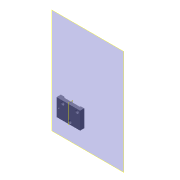
# Autodesk Inventor part: cellSTORM_v5_chiptray_old_0
Saved by Autodesk Inventor 2022 (Build 260153000, 153)
## iProperties
Created: 2020-05-10
Part Number: cellSTORM_v5_chiptray_old_0
Material: Generic
Document SubType Name: Modeling
Designer: diederichbenedict
Density: 1 g/cm^3
Appearance: Default
Author: diederichbenedict
Autodesk Inventor part; units mm, degrees
ref_plane "YZ Plane" through (0, 0, 0) normal (1, 0, 0) x (0, 1, 0)
ref_plane "XZ Plane" through (0, 0, 0) normal (0, 1, 0) x (-1, 0, 0)
ref_plane "XY Plane" through (0, 0, 0) normal (0, 0, 1) x (1, 0, 0)
ref_plane "Work Plane1" through (52.5141, 202.7033, 6.4479) normal (0, 0, -1) x (0, 1, 0)
sketch "Sketch1" plane through (52.5141, 202.7033, 6.4479) normal (0, 0, -1) x (0, 1, 0)
  line L0 (-34.8114, -13.0433) -> (-63.8114, -13.0433)
  line L1 (-63.8114, -13.0433) -> (-63.8114, -52.6244)
  line L2 (-63.8114, -52.6244) -> (-34.8114, -52.6244)
  line L3 (-34.8114, -52.6244) -> (-34.8114, -13.0433)
  circle A0 centre (-59.5444, -32.8338) radius 2.95
  circle A1 centre (-38.8114, -20.7095) radius 2.95
  circle A2 centre (-38.8114, -44.9582) radius 2.95 construction
  line L4 (-60.26, -25.0657) -> (-36.5, -25.0657) construction
  line L5 (-36.5, -25.0657) -> (-36.5, -52.0657) construction
  line L6 (-60.26, -52.0657) -> (-60.26, -25.0657) construction
  line L7 (-57.1632, -22.5233) -> (-33.4032, -22.5233) construction
  line L8 (-33.4032, -22.5233) -> (-33.4032, -49.5233) construction
  line L9 (-33.4032, -49.5233) -> (-57.1632, -49.5233) construction
  line L10 (-57.1632, -49.5233) -> (-57.1632, -22.5233) construction
  circle A3 centre (-38.8114, -44.9582) radius 2.95
  point P0 (-202.7033, -52.5141)
  point P1 (-56.7146, -27.9576)
  point P2 (-25.3114, -32.8338)
  dimension "d4" = 5.9
  dimension "d5" = 5.9
  dimension "d6" = 5.9
  dimension "d37" = 12.1244
  dimension "d38" = 12.1244
  constraints: 22 end point, 5 parallel, 4 centre point, 3 horizontal, 3 perpendicular, 1 coincident, 1 concentric, 1 other
  measures "d4" diameter of A0
  measures "d5" diameter of A1
  measures "d6" diameter of A2
  measures "d37" vertical distance of A1.centre A0.centre
  measures "d38" vertical distance of A2.centre A0.centre
extrude "Extrusion1" add sketch "Sketch1" along normal blind 4
sketch "Sketch2" plane through (52.5141, 202.7033, 2.4479) normal (0, 0, -1) x (-1, 0, 0)
  circle A0 centre (44.9582, -38.8114) radius 2.95 projected
  circle A1 centre (20.7095, -38.8114) radius 2.95 projected
  circle A2 centre (32.8338, -59.5444) radius 2.95 projected
  line L0 (13.0433, -34.8114) -> (13.0433, -63.8114) projected
  line L1 (13.0433, -63.8114) -> (52.6244, -63.8114) projected
  line L2 (52.6244, -63.8114) -> (52.6244, -34.8114) projected
  line L3 (52.6244, -34.8114) -> (13.0433, -34.8114) projected
  point P0 (52.5141, -202.7033)
extrude "Extrusion2" add sketch "Sketch2" along normal blind 1.5 contours A0 | A1 | A2 | L3 L2 L1 L0
sketch "Sketch5" plane through (52.5141, 202.7033, 0.9479) normal (0, 0, -1) x (-1, 0, 0)
  arc A0 (46.5221, -54.1283) -> (46.5221, -43.4579) centre (46.5221, -48.7931) ccw projected
  circle A1 centre (49.353, -48.7931) radius 1.4
  point P0 (52.5141, -202.7033)
  dimension "d30" = 2.8
  constraints: 1 centre point
  measures "d30" diameter of A1
extrude "Extrusion5" cut sketch "Sketch5" against normal through all
equation "\"d31\" = d30"
body "Solid1"
